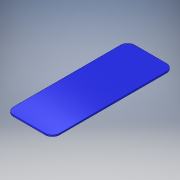
# Autodesk Inventor part: PCB
Saved by Autodesk Inventor 2019 (Build 230136000, 136)
## iProperties
Created: 2020-02-13
Part Number: PCB
Material: Generic
Document SubType Name: Modeling
Designer: close
Density: 1 g/cm^3
Appearance: Blue - Wall Paint - Glossy
Author: close
Autodesk Inventor part; units mm, degrees
ref_plane "YZ Plane" through (0, 0, 0) normal (1, 0, 0) x (0, 1, 0)
ref_plane "XZ Plane" through (0, 0, 0) normal (0, 1, 0) x (-1, 0, 0)
ref_plane "XY Plane" through (0, 0, 0) normal (0, 0, 1) x (1, 0, 0)
sketch "Sketch1" plane through (0, 0, 0) normal (0, 1, 0) x (-1, 0, 0)
  line L0 (0, 0) -> (39.5, 0)
  line L1 (39.5, 0) -> (39.5, -104.35)
  line L2 (39.5, -104.35) -> (0, -104.35)
  line L3 (0, -104.35) -> (0, 0)
  dimension "d0" = 104.35
  dimension "d1" = 39.5
  constraints: 8 end point, 2 parallel, 1 horizontal, 1 perpendicular
  measures "d0" distance of L0.end L1.end
  measures "d1" distance of L1.end L2.end
extrude "Extrusion1" add sketch "Sketch1" along normal blind 1.2
fillet "Fillet1" radius 6 4 edges at (0, 0.6, 0) (-39.5, 0.6, 0) (0, 0.6, -104.35) (-39.5, 0.6, -104.35)
body "Solid1"
